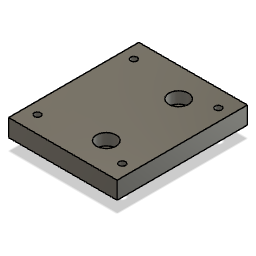
Emergency switch mount v2 (Autodesk Fusion 360 design; units mm, degrees)
Autodesk Fusion 360 part; units mm, degrees
sketch "Sketch1" plane through (0, 0, 0) normal (0, 1, 0) x (1, 0, 0)
  line L0 (29.25, 33.25) -> (-29.25, 33.25)
  line L1 (-29.25, 33.25) -> (-29.25, -33.25)
  line L2 (-29.25, -33.25) -> (29.25, -33.25)
  line L3 (29.25, -33.25) -> (29.25, 33.25)
  line L4 (29.25, 33.25) -> (-29.25, -33.25) construction
  line L5 (-29.25, 33.25) -> (29.25, -33.25) construction
  circle A0 centre (-29.25, -33.25) radius 2.25
  circle A1 centre (29.25, -33.25) radius 2.25
  circle A2 centre (-29.25, 33.25) radius 2.25
  circle A3 centre (29.25, 33.25) radius 2.25
  line L6 (37.5, 45) -> (-37.5, 45)
  line L7 (-37.5, 45) -> (-37.5, -45)
  line L8 (-37.5, -45) -> (37.5, -45)
  line L9 (37.5, -45) -> (37.5, 45)
  line L10 (37.5, 45) -> (-37.5, -45) construction
  line L11 (-37.5, 45) -> (37.5, -45) construction
  dimension "d1" = 58.5
  dimension "d2" = 66.5
  dimension "d3" = 4.5
  dimension "d4" = 4.5
  dimension "d5" = 4.5
  dimension "d6" = 4.5
  dimension "d7" = 75
  dimension "d8" = 90
  constraint horizontal L0
  constraint perpendicular L0 L1
  constraint parallel L0 L2
  constraint parallel L1 L3
  constraint coincident L4 origin
  constraint coincident L5 origin
  constraint coincident L1.end L2.start
  constraint coincident L2.end L3.start
  constraint coincident L0.end L1.start
  constraint coincident L0.start L3.end
  constraint horizontal L6
  constraint perpendicular L6 L7
  constraint parallel L6 L8
  constraint parallel L7 L9
  constraint coincident L10 origin
  constraint coincident L11 origin
  measures "d1" distance of L1.end L2.end
  measures "d2" distance of L0.end L1.end
  measures "d3" diameter of A0
  measures "d4" diameter of A1
  measures "d5" diameter of A2
  measures "d6" diameter of A3
  measures "d7" distance of L7.end L8.end
  measures "d8" distance of L6.end L7.end
extrude "Extrude1" add sketch "Sketch1" along normal blind 12 contours L0 L1 L2 L3 A0 A1 A2 A3 | L6 L7 L8 L9
sketch "Sketch2" plane through (0, 0, 0) normal (0, -1, 0) x (1, 0, 0)
  circle A0 centre (29.25, -33.25) radius 2.25
  circle A1 centre (-29.25, 33.25) radius 2.25
  circle A2 centre (-29.25, -33.25) radius 2.25
  circle A3 centre (29.25, 33.25) radius 2.25
  line L0 (37.5, -45) -> (37.5, 45)
  line L1 (37.5, 45) -> (-37.5, 45)
  line L2 (-37.5, 45) -> (-37.5, -45)
  line L3 (-37.5, -45) -> (37.5, -45)
  line L4 (-35, -30) -> (35, -30)
  line L5 (35, -30) -> (35, 30)
  line L6 (35, 30) -> (-35, 30)
  line L7 (-35, 30) -> (-35, -30)
  line L8 (-35, -30) -> (35, 30) construction
  line L9 (35, -30) -> (-35, 30) construction
  line L10 (-25, -20) -> (-17, -20)
  line L11 (-17, -20) -> (-17, -30)
  line L12 (-17, -30) -> (-25, -30)
  line L13 (-25, -30) -> (-25, -20)
  line L14 (25, -20) -> (17, -20)
  line L15 (17, -20) -> (17, -30)
  line L16 (17, -30) -> (25, -30)
  line L17 (25, -30) -> (25, -20)
  line L18 (25, 20) -> (17, 20)
  line L19 (17, 20) -> (17, 30)
  line L20 (17, 30) -> (25, 30)
  line L21 (25, 30) -> (25, 20)
  line L22 (-25, 20) -> (-17, 20)
  line L23 (-17, 20) -> (-17, 30)
  line L24 (-17, 30) -> (-25, 30)
  line L25 (-25, 30) -> (-25, 20)
  circle A4 centre (10, -25) radius 4.5
  circle A5 centre (-10, -25) radius 4.5
  circle A6 centre (10, 25) radius 4.5
  circle A7 centre (-10, 25) radius 4.5
  dimension "d11" = 60
  dimension "d25" = 8
  dimension "d26" = 8
  dimension "d27" = 8
  dimension "d28" = 8
  dimension "d29" = 9
  dimension "d30" = 9
  dimension "d31" = 9
  dimension "d32" = 9
  constraint horizontal L4
  constraint perpendicular L4 L5
  constraint parallel L4 L6
  constraint parallel L5 L7
  constraint coincident L8 origin
  constraint coincident L9 origin
  constraint horizontal L10
  constraint vertical L11
  constraint horizontal L12
  constraint vertical L13
  constraint horizontal L14
  constraint vertical L15
  constraint horizontal L16
  constraint vertical L17
  constraint horizontal L18
  constraint vertical L19
  constraint horizontal L20
  constraint vertical L21
  constraint horizontal L22
  constraint vertical L23
  constraint horizontal L24
  constraint vertical L25
  measures "d11" distance of L4.end L5.end
  measures "d25" distance of L10.start L10.end
  measures "d26" distance of L14.start L14.end
  measures "d27" distance of L18.start L18.end
  measures "d28" distance of L22.start L22.end
  measures "d29" diameter of A4
  measures "d30" diameter of A5
  measures "d31" diameter of A6
  measures "d32" diameter of A7
extrude "Extrude2" add sketch "Sketch2" along normal blind 8 contours L4 L10 L11 L12 L13 | L6 L22 L23 L24 L25 | L4 L14 L15 L16 L17 | L6 L18 L19 L20 L21
sketch "Sketch3" plane through (0, 0, 0) normal (0, -1, 0) x (1, 0, 0)
  line L0 (-25, 30) -> (-17, 30)
  line L1 (25, -30) -> (17, -30)
  line L2 (37.5, -45) -> (37.5, 45)
  line L3 (-37.5, 45) -> (-37.5, -45)
  line L4 (-17, 30) -> (-17, 20)
  line L5 (-17, 20) -> (-25, 20)
  line L6 (-25, 20) -> (-25, 30)
  line L7 (17, -30) -> (17, -20)
  line L8 (17, -20) -> (25, -20)
  line L9 (25, -20) -> (25, -30)
  line L10 (25, 30) -> (25, 20)
  line L11 (25, 20) -> (17, 20)
  line L12 (17, 20) -> (17, 30)
  line L13 (17, 30) -> (25, 30)
  line L14 (-25, -30) -> (-25, -20)
  line L15 (-25, -20) -> (-17, -20)
  line L16 (-17, -20) -> (-17, -30)
  line L17 (-17, -30) -> (-25, -30)
  line L18 (37.5, 45) -> (-37.5, 45)
  line L19 (-37.5, -45) -> (37.5, -45)
  circle A0 centre (29.25, 33.25) radius 2.25
  circle A1 centre (29.25, -33.25) radius 2.25
  circle A2 centre (-29.25, 33.25) radius 2.25
  circle A3 centre (-29.25, -33.25) radius 2.25
  circle A4 centre (29.25, -33.25) radius 5.25
  circle A5 centre (-29.25, -33.25) radius 5.25
  circle A6 centre (-29.25, 33.25) radius 5.25
  circle A7 centre (29.25, 33.25) radius 5.25
  dimension "d41" = 10.5
  dimension "d42" = 10.5
  dimension "d43" = 10.5
  dimension "d44" = 10.5
  constraint concentric A1 A4
  constraint concentric A3 A5
  constraint concentric A2 A6
  constraint concentric A0 A7
  measures "d41" diameter of A4
  measures "d42" diameter of A5
  measures "d43" diameter of A6
  measures "d44" diameter of A7
sketch "Sketch4" plane through (0, 0, 0) normal (0, -1, 0) x (1, 0, 0)
  line L0 (-37.5, 45) -> (-37.5, -45)
  line L1 (25, -30) -> (17, -30)
  line L2 (17, 30) -> (25, 30)
  line L3 (-37.5, -45) -> (37.5, -45)
  line L4 (17, -30) -> (17, -20)
  line L5 (17, -20) -> (25, -20)
  line L6 (25, -20) -> (25, -30)
  line L7 (25, 30) -> (25, 20)
  line L8 (25, 20) -> (17, 20)
  line L9 (17, 20) -> (17, 30)
  line L10 (37.5, -45) -> (37.5, 45)
  line L11 (37.5, 45) -> (-37.5, 45)
  line L12 (-17, 30) -> (-17, 20)
  line L13 (-17, 20) -> (-25, 20)
  line L14 (-25, 20) -> (-25, 30)
  line L15 (-25, -30) -> (-25, -20)
  line L16 (-25, -20) -> (-17, -20)
  line L17 (-17, -20) -> (-17, -30)
  line L18 (-17, -30) -> (-25, -30)
  line L19 (-25, 30) -> (-17, 30)
  circle A0 centre (29.25, 33.25) radius 2.25
  circle A1 centre (-29.25, 33.25) radius 2.25
  circle A2 centre (-29.25, -33.25) radius 2.25
  circle A3 centre (29.25, -33.25) radius 2.25
sketch "Sketch5" plane through (0, 12, 0) normal (0, 1, 0) x (-1, 0, 0)
  circle A0 centre (-29.25, 33.25) radius 2.25
  circle A1 centre (-29.25, -33.25) radius 2.25
  circle A2 centre (29.25, 33.25) radius 2.25
  circle A3 centre (29.25, -33.25) radius 2.25
  line L0 (-37.5, 45) -> (-37.5, -45)
  line L1 (-37.5, -45) -> (37.5, -45)
  line L2 (37.5, -45) -> (37.5, 45)
  line L3 (37.5, 45) -> (-37.5, 45)
  circle A4 centre (10, -25) radius 6.75
  circle A5 centre (-10, -25) radius 6.75
  circle A6 centre (10, 25) radius 6.75
  circle A7 centre (-10, 25) radius 6.75
  dimension "d33" = 13.5
  dimension "d34" = 13.5
  dimension "d35" = 13.5
  dimension "d36" = 13.5
  measures "d33" diameter of A4
  measures "d34" diameter of A5
  measures "d35" diameter of A6
  measures "d36" diameter of A7
extrude "Extrude4" cut sketch "Sketch5" against normal blind 8 contours A5 | A7
extrude "Extrude5" cut sketch "Sketch2" against normal blind 16 contours A4 | A6
extrude "Extrude6" cut sketch "Sketch3" against normal blind 5 contours A4 | A5 | A6 | A7
